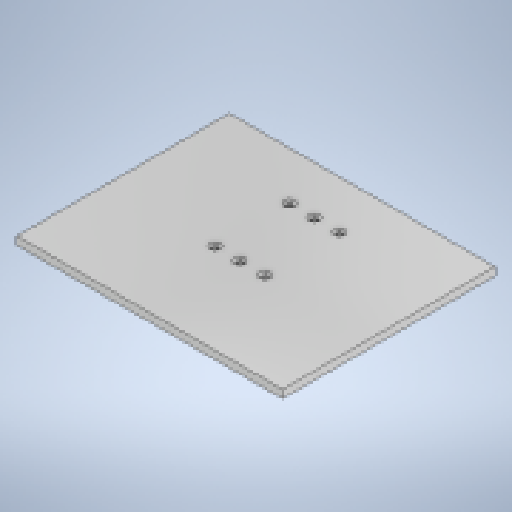
# Autodesk Inventor part: axis_12_bottom_frame(bottom)
Saved by Autodesk Inventor 2025.2 (Build 292293000, 293)
## iProperties
Created: 2025-05-04
Part Number: axis_12_bottom_frame(bottom)
Material: Aluminum 6061-AHC
Document SubType Name: Sheet Metal
Designer: User
Density: 2.7 g/cm^3
Sheet Metal Rule: Default_mm
Appearance: Aluminum - Dark
Author: User
Autodesk Inventor part; units mm, degrees
ref_plane "YZ Plane" through (0, 0, 0) normal (1, 0, 0) x (0, 1, 0)
ref_plane "XZ Plane" through (0, 0, 0) normal (0, 1, 0) x (-1, 0, 0)
ref_plane "XY Plane" through (0, 0, 0) normal (0, 0, 1) x (1, 0, 0)
sketch "Sketch1" plane through (0, 0, 0) normal (0, 1, 0) x (-1, 0, 0)
  line L0 (50, -12) -> (-50, -12)
  line L1 (-50, -12) -> (-50, 68)
  line L2 (-50, 68) -> (50, 68)
  line L3 (50, 68) -> (50, -12)
  point P0 (0, 0)
  dimension "d0" = 100
  dimension "d1" = 80
  dimension "d2" = 12
  dimension "d3" = 50
  measures "d0" distance of L0.start L0.end
  measures "d1" distance of L0.end L1.end
  measures "d2" distance from line of L0 point (0, 0)
  measures "d3" distance from line of point (0, 0) L3
extrude "Plate1" add sketch "Sketch1" along normal blind 3
sketch "Sketch3" plane through (0, 3, 0) normal (0, 1, 0) x (1, 0, 0)
  circle A0 centre (9.405, -34) radius 1.05 projected
  circle A1 centre (9.405, -6) radius 1.05 projected
  circle A2 centre (0, -34) radius 1.05 projected
  circle A3 centre (0, -6) radius 1.05 projected
  circle A4 centre (-9.405, -34) radius 1.05 projected
  circle A5 centre (-9.405, -6) radius 1.05 projected
  line L0 (15.405, 0) -> (15.405, -40) projected
  line L1 (-15.405, -40) -> (15.405, -40) projected
  line L2 (-15.405, -40) -> (-15.405, 0) projected
  line L3 (15.405, 0) -> (-15.405, 0) projected
  point P0 (0, 0)
  constraints: 1 other
hole "Hole1" at (-9.405, 3, 6) at (0, 3, 6) at (9.405, 3, 6) at (9.405, 3, 34) at (0, 3, 34) at (-9.405, 3, 34) direction (0, -1, 0) diameter 2.1 depth 3 countersink diameter 4 countersink angle 90
equation "\"d20\" = Thickness"
equation "\"d4\" = Thickness"
equation "\"BendReliefWidth\" = Thickness"
equation "\"BendReliefDepth\" = 0.5 * Thickness"
equation "\"CornerReliefSize\" = 4 * Thickness"
equation "\"MinimumRemnant\" = 2 * Thickness"
equation "\"TransitionRadius\" = BendRadius"
equation "\"JacobiRadiusSize\" = BendRadius"
equation "\"GapSize\" = Thickness"
equation "\"Thickness\" = 3"
equation "\"BendRadius\" = 0.31"
body "Solid1"
